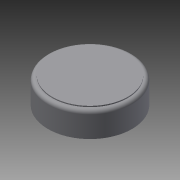
# Autodesk Inventor part: Battery
Saved by Autodesk Inventor 2013 (Build 170138000, 138)
## iProperties
Created: 2014-07-07
Part Number: Battery
Material: Genérico
Document SubType Name: Chapa
Designer: Administrador
Density: 1 g/cm^3
Sheet Metal Rule: Por defecto_mm
Author: Administrador
Autodesk Inventor part; units mm, degrees
ref_plane "YZ Plane" through (0, 0, 0) normal (1, 0, 0) x (0, 1, 0)
ref_plane "XZ Plane" through (0, 0, 0) normal (0, 1, 0) x (-1, 0, 0)
ref_plane "XY Plane" through (0, 0, 0) normal (0, 0, 1) x (1, 0, 0)
sketch "Boceto1" plane through (0, 0, 0) normal (0, 0, 1) x (1, 0, 0)
  circle A0 centre (0, 0) radius 12.25
  dimension "d0" = 24.5
  constraints: 1 centre point
  measures "d0" diameter of A0
extrude "Extrusión1" add sketch "Boceto1" along normal blind 7.2
sketch "Boceto2" plane through (0, 0, 7.2) normal (0, 0, 1) x (1, 0, 0)
  circle A0 centre (0, 0) radius 11
  dimension "d3" = 22
  constraints: 1 centre point
  measures "d3" diameter of A0
extrude "Extrusión2" add sketch "Boceto2" along normal blind 0.3
fillet "Empalme1" radius 1 1 edges at (-12.25, 0, 7.2)
equation "\"Radio_pliegue\" = Grosor"
equation "\"Anchura_desahogo_plegado\" = Grosor"
equation "\"Profundidad_desahogo_plegado\" = 0.5 * Grosor"
equation "\"Tamaño_destalonado\" = 4 * Grosor"
equation "\"Remanente_mínimo\" = 2 * Grosor"
equation "\"Radiodetransición\" = Radio_pliegue"
equation "\"Tamaño_de_radio_de_Jacobi\" = Radio_pliegue"
equation "\"TamañoSeparación\" = Grosor"
equation "\"Grosor\" = 0.5"
